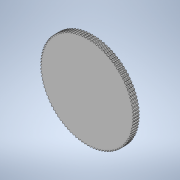
# Autodesk Inventor part: TimingPulley_S5M_Template
Saved by Autodesk Inventor 2021 (Build 250183000, 183)
## iProperties
Created: 2021-03-01
Part Number: TimingPulley_S5M_Template
Material: 一般
Document SubType Name: Modeling
Designer: yuta2
Density: 1 g/cm^3
Appearance: 既定
Author: yuta2
Autodesk Inventor part; units mm, degrees
ref_plane "YZ Plane" through (0, 0, 0) normal (1, 0, 0) x (0, 1, 0)
ref_plane "XZ Plane" through (0, 0, 0) normal (0, 1, 0) x (-1, 0, 0)
ref_plane "XY Plane" through (0, 0, 0) normal (0, 0, 1) x (1, 0, 0)
sketch "スケッチ1" plane through (0, 0, 0) normal (0, 0, 1) x (1, 0, 0)
  circle A0 centre (0, 0) radius 79.5775
  circle A1 centre (0, 0) radius 80.1275
  dimension "d0" = 159.155
  dimension "d1" = 160.255
  constraints: 2 centre point, 2 coincident
  measures "d0" diameter of A0
  measures "d1" diameter of A1
extrude "押し出し1" add sketch "スケッチ1" along normal blind 10 contours A0 | A1
sketch "スケッチ2" plane through (0, 0, 10) normal (0, 0, 1) x (1, 0, 0)
  circle A0 centre (0, 0) radius 79.5775
  circle A1 centre (0, 0) radius 80.1275
  circle A2 centre (0, 0) radius 78.3575
  line L0 (0, 0) -> (0, 80.1275) construction
  circle A3 centre (0, 0) radius 80.1275 projected
  line L1 (0, 0) -> (3.2716, 80.0607) construction
  circle A4 centre (0, 0) radius 80.6275
  arc A5 (2.4068, 78.4065) -> (3.1278, 79.6566) centre (0, 80.6275) ccw
  arc A6 (0.1271, 79.7179) -> (0.7965, 78.4394) centre (3.292, 80.5603) ccw
  arc A7 (0.7965, 78.4394) -> (0.9838, 78.3513) centre (0.987, 78.6013) ccw
  arc A8 (2.216, 78.3261) -> (2.4068, 78.4065) centre (2.2231, 78.576) ccw
  arc A9 (0.1271, 79.7179) -> (-0.4071, 80.1265) centre (-0.4044, 79.5765) ccw
  arc A10 (3.6783, 80.043) -> (3.1278, 79.6566) centre (3.6531, 79.4936) ccw
  circle A11 centre (0, 0) radius 80.1275 projected
  dimension "d4" = 159.155
  dimension "d5" = 160.255
  dimension "d6" = 156.715
  dimension "d7" = 2.34
  dimension "d9" = 161.255
  dimension "d10" = 3.275
  dimension "d11" = 3.275
  dimension "d12" = 0.25
  dimension "d13" = 0.25
  dimension "d14" = 0.55
  dimension "d15" = 0.55
  constraints: 27 point on circle, 10 centre point, 8 tangent, 4 coincident, 4 end point, 2 point on line, 1 vertical
  measures "d4" diameter of A0
  measures "d5" diameter of A1
  measures "d6" diameter of A2
  measures "d7" angle of L1 L0
  measures "d9" diameter of A4
  measures "d10" radius of A5
  measures "d11" radius of A6
  measures "d12" radius of A7
  measures "d13" radius of A8
  measures "d14" radius of A9
  measures "d15" radius of A10
extrude "押し出し2" cut sketch "スケッチ2" against normal through all contours A5 A8 A2 A7 A6 A0 | A0 A6 A9 A1 A10 A5 picked at (1.685, 79.1519) picked at (1.7942, 79.9218)
pattern_circular "円形状パターン1" count 100 over 360 about axis through (0, 0, 0) along (0, 0, 1) of "押し出し2"
equation "\"d0\" = PD"
equation "\"d2\" = t"
equation "\"d4\" = PD"
equation "\"PD\" = 1.59155 * z"
equation "\"t\" = 10"
equation "\"z\" = 100"
